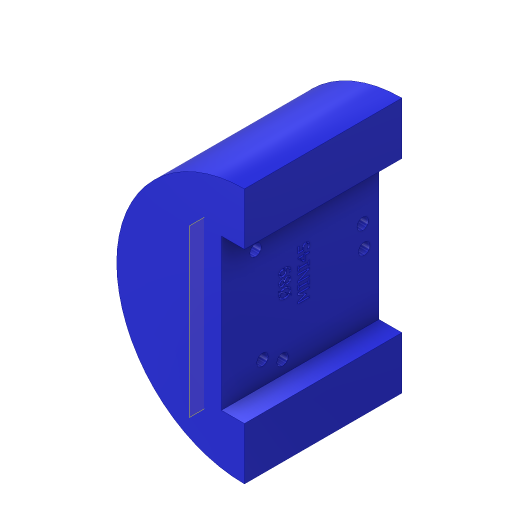
# Autodesk Inventor part: MINI45NewShell89_B
Saved by Autodesk Inventor 2023 (Build 270158000, 158)
## iProperties
Created: 2016-07-01
Part Number: MINI45NewShell89_B
Material: ABS Plastic
Document SubType Name: Modeling
Designer: Administrateur
Density: 1.06 g/cm^3
Appearance: Blue - Wall Paint - Glossy
Author: Administrateur
Autodesk Inventor part; units mm, degrees
ref_plane "XZ Plane" through (0, 0, 0) normal (0, 1, 0) x (-1, 0, 0)
sketch "Sketch1" plane through (0, 0, 0) normal (0, 0, 1) x (1, 0, 0)
  arc A0 (0, 38.9636) -> (0, -38.9636) centre (0, 0) ccw
  line L0 (0, 38.9636) -> (0, 23)
  line L1 (0, 23) -> (-7, 23)
  line L2 (-7, 23) -> (-7, 0)
  line L3 (-46.5484, 0) -> (26.4312, 0) construction
  line L4 (0, -38.9636) -> (0, -23)
  line L5 (0, -23) -> (-7, -23)
  line L6 (-7, -23) -> (-7, 0)
  dimension "d2" = 38.9636
  dimension "d3" = 46
  dimension "d4" = 7
  dimension "d27" = 23
  dimension "d28" = 15.9636
  constraints: 14 end point, 2 horizontal, 2 point on circle, 2 symmetric about line, 1 centre point, 1 coincident, 1 perpendicular, 1 vertical
  measures "d2" radius of A0
  measures "d3" distance between parallel lines of L5 L1
  measures "d4" distance of L0.end L1.end
  measures "d27" distance of L1.end L2.end
  measures "d28" distance of L0.start L0.end
extrude "Extrusion1" add sketch "Sketch1" along normal blind 48
sketch "Sketch2" plane through (-7, -23, 0) normal (1, 0, 0) x (0, 0, -1)
  line L0 (-24, 23) -> (-48, 23) construction
  line L1 (-48, 61.9636) -> (-48, -15.9636) construction
  line L2 (0, 61.9636) -> (-48, 61.9636) construction
  line L3 (-24, 61.9636) -> (-24, -15.9636) construction
  line L4 (0, -15.9636) -> (-48, -15.9636) construction
  line L5 (-24, 23) -> (-37.6292, 37.1134) construction
  circle A0 centre (-24, 23) radius 19.62 construction
  line L6 (-24, 23) -> (-31.9802, 40.9238) construction
  line L7 (-24, 23) -> (-29.408, 4.14) construction
  line L8 (-24, 23) -> (-35.5323, 7.1271) construction
  line L9 (-24, 23) -> (-4.9628, 27.7465) construction
  line L10 (-24, 23) -> (-4.4875, 20.9492) construction
  point P0 (0, 23)
  dimension "d32" = 39.24
  dimension "d34" = 20
  dimension "d37" = 360
  dimension "d39" = 66
  constraints: 16 end point, 11 coincident, 4 midpoint, 2 point on circle, 1 centre point, 17 other
  measures "d32" diameter of A0
  measures "d34" angle of L5 L6
  measures "d39" angle of L0 L6
hole "Hole1" at (-7, 17.9238, 31.9802) at (-7, 14.1134, 37.6292) at (-7, -15.8729, 35.5323) at (-7, -18.86, 29.408) at (-7, -2.0508, 4.4875) at (-7, 4.7465, 4.9628) direction (-1, 0, 0) diameter 3.5 end through all
ref_plane "Work Plane1" through (-38.9636, 0, 0) normal (1, 0, 0) x (0, 1, 0)
ref_plane "Work Plane2" through (-10, 0, 0) normal (1, 0, 0) x (0, 1, 0)
ref_plane "Work Plane3" through (-12.3, -23, 0) normal (1, 0, 0) x (0, 0, -1)
sketch "Sketch4" plane through (-12.3, -23, 0) normal (1, 0, 0) x (0, 0, -1)
  line L0 (0, 61.9636) -> (0, -15.9636) projected
  line L1 (0, -15.9636) -> (-48, -15.9636) projected
  line L2 (-48, 61.9636) -> (-48, -15.9636) projected
  line L3 (0, 61.9636) -> (-48, 61.9636) projected
  circle A0 centre (-31.9802, 40.9238) radius 1.75 projected
  circle A1 centre (-37.6292, 37.1134) radius 1.75 projected
  circle A2 centre (-35.5323, 7.1271) radius 1.75 projected
  circle A3 centre (-29.408, 4.14) radius 1.75 projected
  circle A4 centre (-4.4875, 20.9492) radius 1.75 projected
  circle A5 centre (-4.9628, 27.7465) radius 1.75 projected
  point P0 (0, 23)
  point P1 (-4.4875, 22.6992)
  point P2 (-35.5323, 8.8771)
  point P3 (-31.9802, 42.6738)
  point P4 (-37.6292, 38.8634)
  point P5 (-29.408, 5.89)
  point P6 (-4.9628, 29.4965)
  constraints: 6 coincident, 6 vertical alignment, 6 other
hole "Hole3" at (-12.3, 17.9238, 31.9802) at (-12.3, 14.1134, 37.6292) at (-12.3, -15.8729, 35.5323) at (-12.3, -18.86, 29.408) at (-12.3, -2.0508, 4.4875) at (-12.3, 4.7465, 4.9628) direction (-1, 0, 0) diameter 6.5 end through all
sketch "Sketch6" plane through (-7, -23, 0) normal (1, 0, 0) x (0, 0, -1)
  line L0 (-30.6568, 16.0385) -> (-30.6568, 31.8055) construction
  line L1 (-30.6568, 31.8055) -> (-15.416, 31.8055) construction
  line L2 (-15.416, 31.8055) -> (-15.416, 16.0385) construction
  line L3 (-15.416, 16.0385) -> (-30.6568, 16.0385) construction
  spline S0 degree 2 poles (-28.6913, 22.8428) (-27.8234, 22.8428) (-26.8675, 21.9976) (-26.8675, 21.2942) knots 0 0 0 1 2 2 2
  spline S1 degree 2 poles (-26.8675, 21.2942) (-26.8675, 21.0361) (-27.0037, 20.5908) (-27.1285, 20.4121) knots 0 0 0 1 2 2 2
  line L4 (-27.1285, 20.4121) -> (-26.669, 20.1001)
  line L5 (-26.669, 20.1001) -> (-26.669, 19.7541)
  line L6 (-26.669, 19.7541) -> (-27.3213, 20.1965)
  spline S2 degree 2 poles (-27.3213, 20.1965) (-27.5539, 19.9866) (-28.2403, 19.7484) (-28.6913, 19.7484) knots 0 0 0 1 2 2 2
  spline S3 degree 2 poles (-28.6913, 19.7484) (-29.5563, 19.7484) (-30.515, 20.5964) (-30.515, 21.2942) knots 0 0 0 1 2 2 2
  spline S4 degree 2 poles (-30.515, 21.2942) (-30.515, 21.5636) (-30.3846, 21.9834) (-30.2569, 22.1706) knots 0 0 0 1 2 2 2
  line L7 (-30.2569, 22.1706) -> (-30.6568, 22.44)
  line L8 (-30.6568, 22.44) -> (-30.6568, 22.7889)
  line L9 (-30.6568, 22.7889) -> (-30.0669, 22.3862)
  spline S5 degree 2 poles (-30.0669, 22.3862) (-29.8343, 22.6017) (-29.1593, 22.8428) (-28.6913, 22.8428) knots 0 0 0 1 2 2 2
  spline S6 degree 2 poles (-28.6913, 22.3635) (-29.0146, 22.3635) (-29.5223, 22.233) (-29.6897, 22.1252) knots 0 0 0 1 2 2 2
  line L10 (-29.6897, 22.1252) -> (-27.4858, 20.6503)
  spline S7 degree 2 poles (-27.4858, 20.6503) (-27.3781, 20.7836) (-27.2703, 21.0843) (-27.2703, 21.297) knots 0 0 0 1 2 2 2
  spline S8 degree 2 poles (-27.2703, 21.297) (-27.2703, 21.782) (-28.0021, 22.3635) (-28.6913, 22.3635) knots 0 0 0 1 2 2 2
  spline S9 degree 2 poles (-29.9024, 21.9323) (-30.0073, 21.8104) (-30.1123, 21.4899) (-30.1123, 21.297) knots 0 0 0 1 2 2 2
  spline S10 degree 2 poles (-30.1123, 21.297) (-30.1123, 20.8092) (-29.389, 20.2277) (-28.6913, 20.2277) knots 0 0 0 1 2 2 2
  spline S11 degree 2 poles (-28.6913, 20.2277) (-28.3736, 20.2277) (-27.8801, 20.3497) (-27.7042, 20.4603) knots 0 0 0 1 2 2 2
  line L11 (-27.7042, 20.4603) -> (-29.9024, 21.9323)
  spline S12 degree 2 poles (-26.8619, 24.312) (-26.8619, 24.0511) (-27.0179, 23.6228) (-27.1625, 23.4725) knots 0 0 0 1 2 2 2
  spline S13 degree 2 poles (-27.1625, 23.4725) (-27.3043, 23.325) (-27.6901, 23.1718) (-27.9085, 23.1718) knots 0 0 0 1 2 2 2
  spline S14 degree 2 poles (-27.9085, 23.1718) (-28.1921, 23.1718) (-28.6686, 23.4753) (-28.8104, 23.7646) knots 0 0 0 1 2 2 2
  line L12 (-28.8104, 23.7646) -> (-28.8246, 23.7646)
  spline S15 degree 2 poles (-28.8246, 23.7646) (-28.9749, 23.5065) (-29.3323, 23.2569) (-29.5989, 23.2569) knots 0 0 0 1 2 2 2
  spline S16 degree 2 poles (-29.5989, 23.2569) (-29.9931, 23.2569) (-30.5207, 23.8525) (-30.5207, 24.312) knots 0 0 0 1 2 2 2
  spline S17 degree 2 poles (-30.5207, 24.312) (-30.5207, 24.7885) (-30.0215, 25.3643) (-29.6301, 25.3643) knots 0 0 0 1 2 2 2
  spline S18 degree 2 poles (-29.6301, 25.3643) (-29.3947, 25.3643) (-28.9352, 25.0891) (-28.8047, 24.831) knots 0 0 0 1 2 2 2
  line L13 (-28.8047, 24.831) -> (-28.7905, 24.831)
  spline S19 degree 2 poles (-28.7905, 24.831) (-28.6487, 25.1374) (-28.2403, 25.4522) (-27.917, 25.4522) knots 0 0 0 1 2 2 2
  spline S20 degree 2 poles (-27.917, 25.4522) (-27.4688, 25.4522) (-26.8619, 24.7998) (-26.8619, 24.312) knots 0 0 0 1 2 2 2
  spline S21 degree 2 poles (-27.8716, 24.97) (-28.0871, 24.97) (-28.3424, 24.7998) (-28.4729, 24.5588) knots 0 0 0 1 2 2 2
  spline S22 degree 2 poles (-28.4729, 24.5588) (-28.5183, 24.4793) (-28.6232, 24.2127) (-28.6913, 24.0454) knots 0 0 0 1 2 2 2
  spline S23 degree 2 poles (-28.6913, 24.0454) (-28.5636, 23.8525) (-28.1836, 23.6455) (-27.9425, 23.6455) knots 0 0 0 1 2 2 2
  spline S24 degree 2 poles (-27.9425, 23.6455) (-27.6248, 23.6455) (-27.2107, 24.0284) (-27.2107, 24.3177) knots 0 0 0 1 2 2 2
  spline S25 degree 2 poles (-27.2107, 24.3177) (-27.2107, 24.6126) (-27.5653, 24.97) (-27.8716, 24.97) knots 0 0 0 1 2 2 2
  spline S26 degree 2 poles (-29.6244, 24.9048) (-29.8598, 24.9048) (-30.1747, 24.59) (-30.1747, 24.3092) knots 0 0 0 1 2 2 2
  spline S27 degree 2 poles (-30.1747, 24.3092) (-30.1747, 24.0539) (-29.8939, 23.7277) (-29.6528, 23.7277) knots 0 0 0 1 2 2 2
  spline S28 degree 2 poles (-29.6528, 23.7277) (-29.4798, 23.7277) (-29.2387, 23.8951) (-29.1422, 24.0624) knots 0 0 0 1 2 2 2
  spline S29 degree 2 poles (-29.1422, 24.0624) (-29.1025, 24.1333) (-28.9636, 24.434) (-28.9239, 24.5559) knots 0 0 0 1 2 2 2
  spline S30 degree 2 poles (-28.9239, 24.5559) (-29.0798, 24.7601) (-29.4117, 24.9048) (-29.6244, 24.9048) knots 0 0 0 1 2 2 2
  spline S31 degree 2 poles (-29.3039, 25.784) (-29.5734, 25.784) (-30.0215, 25.9599) (-30.1832, 26.1131) knots 0 0 0 1 2 2 2
  spline S32 degree 2 poles (-30.1832, 26.1131) (-30.3392, 26.2577) (-30.5122, 26.6803) (-30.5122, 26.8959) knots 0 0 0 1 2 2 2
  spline S33 degree 2 poles (-30.5122, 26.8959) (-30.5122, 27.137) (-30.3505, 27.5284) (-30.1974, 27.673) knots 0 0 0 1 2 2 2
  spline S34 degree 2 poles (-30.1974, 27.673) (-30.0045, 27.8545) (-29.3805, 28.0531) (-28.9012, 28.0531) knots 0 0 0 1 2 2 2
  spline S35 degree 2 poles (-28.9012, 28.0531) (-28.4672, 28.0531) (-27.6901, 27.8574) (-27.432, 27.6673) knots 0 0 0 1 2 2 2
  spline S36 degree 2 poles (-27.432, 27.6673) (-27.1597, 27.466) (-26.8732, 26.8987) (-26.8732, 26.4846) knots 0 0 0 1 2 2 2
  spline S37 degree 2 poles (-26.8732, 26.4846) (-26.8732, 26.391) (-26.8931, 26.1783) (-26.9214, 26.0875) knots 0 0 0 1 2 2 2
  line L14 (-26.9214, 26.0875) -> (-27.3724, 26.0875)
  line L15 (-27.3724, 26.0875) -> (-27.3724, 26.1102)
  spline S38 degree 2 poles (-27.3724, 26.1102) (-27.3384, 26.1698) (-27.2788, 26.4194) (-27.2788, 26.547) knots 0 0 0 1 2 2 2
  spline S39 degree 2 poles (-27.2788, 26.547) (-27.2788, 27.0065) (-27.8858, 27.5312) (-28.4474, 27.5681) knots 0 0 0 1 2 2 2
  spline S40 degree 2 poles (-28.4474, 27.5681) (-28.3197, 27.3809) (-28.2034, 27.0405) (-28.2034, 26.8391) knots 0 0 0 1 2 2 2
  spline S41 degree 2 poles (-28.2034, 26.8391) (-28.2034, 26.6463) (-28.2885, 26.3258) (-28.4105, 26.1641) knots 0 0 0 1 2 2 2
  spline S42 degree 2 poles (-28.4105, 26.1641) (-28.5551, 25.9769) (-28.9948, 25.784) (-29.3039, 25.784) knots 0 0 0 1 2 2 2
  spline S43 degree 2 poles (-29.0061, 27.5794) (-29.3606, 27.5794) (-29.8088, 27.449) (-29.9307, 27.3327) knots 0 0 0 1 2 2 2
  spline S44 degree 2 poles (-29.9307, 27.3327) (-30.0442, 27.2306) (-30.1293, 27.0178) (-30.1293, 26.893) knots 0 0 0 1 2 2 2
  spline S45 degree 2 poles (-30.1293, 26.893) (-30.1293, 26.6037) (-29.7152, 26.2605) (-29.3238, 26.2605) knots 0 0 0 1 2 2 2
  spline S46 degree 2 poles (-29.3238, 26.2605) (-29.1025, 26.2605) (-28.8161, 26.374) (-28.714, 26.4988) knots 0 0 0 1 2 2 2
  spline S47 degree 2 poles (-28.714, 26.4988) (-28.6402, 26.5896) (-28.592, 26.8136) (-28.592, 26.9441) knots 0 0 0 1 2 2 2
  spline S48 degree 2 poles (-28.592, 26.9441) (-28.592, 27.0944) (-28.6969, 27.4404) (-28.7849, 27.5709) knots 0 0 0 1 2 2 2
  spline S49 degree 2 poles (-28.7849, 27.5709) (-28.8189, 27.5738) (-28.9352, 27.5794) (-29.0061, 27.5794) knots 0 0 0 1 2 2 2
  line L16 (-21.1786, 19.3938) -> (-21.1786, 18.9287)
  line L17 (-21.1786, 18.9287) -> (-24.1936, 18.9287)
  line L18 (-24.1936, 18.9287) -> (-22.143, 18.0154)
  line L19 (-22.143, 18.0154) -> (-22.143, 17.7318)
  line L20 (-22.143, 17.7318) -> (-24.1936, 16.827)
  line L21 (-24.1936, 16.827) -> (-21.1786, 16.827)
  line L22 (-21.1786, 16.827) -> (-21.1786, 16.393)
  line L23 (-21.1786, 16.393) -> (-24.6786, 16.393)
  line L24 (-24.6786, 16.393) -> (-24.6786, 17.0284)
  line L25 (-24.6786, 17.0284) -> (-22.7301, 17.902)
  line L26 (-22.7301, 17.902) -> (-24.6786, 18.7472)
  line L27 (-24.6786, 18.7472) -> (-24.6786, 19.3938)
  line L28 (-24.6786, 19.3938) -> (-21.1786, 19.3938)
  line L29 (-21.1786, 21.3225) -> (-21.1786, 19.9668)
  line L30 (-21.1786, 19.9668) -> (-21.536, 19.9668)
  line L31 (-21.536, 19.9668) -> (-21.536, 20.4121)
  line L32 (-21.536, 20.4121) -> (-24.3212, 20.4121)
  line L33 (-24.3212, 20.4121) -> (-24.3212, 19.9668)
  line L34 (-24.3212, 19.9668) -> (-24.6786, 19.9668)
  line L35 (-24.6786, 19.9668) -> (-24.6786, 21.3225)
  line L36 (-24.6786, 21.3225) -> (-24.3212, 21.3225)
  line L37 (-24.3212, 21.3225) -> (-24.3212, 20.8772)
  line L38 (-24.3212, 20.8772) -> (-21.536, 20.8772)
  line L39 (-21.536, 20.8772) -> (-21.536, 21.3225)
  line L40 (-21.536, 21.3225) -> (-21.1786, 21.3225)
  line L41 (-21.1786, 24.4028) -> (-21.1786, 23.8809)
  line L42 (-21.1786, 23.8809) -> (-24.1964, 22.3323)
  line L43 (-24.1964, 22.3323) -> (-21.1786, 22.3323)
  line L44 (-21.1786, 22.3323) -> (-21.1786, 21.8983)
  line L45 (-21.1786, 21.8983) -> (-24.6786, 21.8983)
  line L46 (-24.6786, 21.8983) -> (-24.6786, 22.5592)
  line L47 (-24.6786, 22.5592) -> (-21.9075, 23.9688)
  line L48 (-21.9075, 23.9688) -> (-24.6786, 23.9688)
  line L49 (-24.6786, 23.9688) -> (-24.6786, 24.4028)
  line L50 (-24.6786, 24.4028) -> (-21.1786, 24.4028)
  line L51 (-21.1786, 26.3314) -> (-21.1786, 24.9757)
  line L52 (-21.1786, 24.9757) -> (-21.536, 24.9757)
  line L53 (-21.536, 24.9757) -> (-21.536, 25.421)
  line L54 (-21.536, 25.421) -> (-24.3212, 25.421)
  line L55 (-24.3212, 25.421) -> (-24.3212, 24.9757)
  line L56 (-24.3212, 24.9757) -> (-24.6786, 24.9757)
  line L57 (-24.6786, 24.9757) -> (-24.6786, 26.3314)
  line L58 (-24.6786, 26.3314) -> (-24.3212, 26.3314)
  line L59 (-24.3212, 26.3314) -> (-24.3212, 25.8861)
  line L60 (-24.3212, 25.8861) -> (-21.536, 25.8861)
  line L61 (-21.536, 25.8861) -> (-21.536, 26.3314)
  line L62 (-21.536, 26.3314) -> (-21.1786, 26.3314)
  line L63 (-22.3812, 29.06) -> (-22.3812, 28.643)
  line L64 (-22.3812, 28.643) -> (-21.1786, 28.643)
  line L65 (-21.1786, 28.643) -> (-21.1786, 28.1921)
  line L66 (-21.1786, 28.1921) -> (-22.3812, 28.1921)
  line L67 (-22.3812, 28.1921) -> (-22.3812, 26.6463)
  line L68 (-22.3812, 26.6463) -> (-22.8747, 26.6463)
  line L69 (-22.8747, 26.6463) -> (-24.6786, 28.2119)
  line L70 (-24.6786, 28.2119) -> (-24.6786, 28.643)
  line L71 (-24.6786, 28.643) -> (-22.7584, 28.643)
  line L72 (-22.7584, 28.643) -> (-22.7584, 29.06)
  line L73 (-22.7584, 29.06) -> (-22.3812, 29.06)
  line L74 (-22.7584, 28.1921) -> (-24.1255, 28.1921)
  line L75 (-24.1255, 28.1921) -> (-22.7584, 27.015)
  line L76 (-22.7584, 27.015) -> (-22.7584, 28.1921)
  spline S50 degree 2 poles (-22.2905, 31.5559) (-22.038, 31.5559) (-21.6069, 31.3943) (-21.4481, 31.2468) knots 0 0 0 1 2 2 2
  spline S51 degree 2 poles (-21.4481, 31.2468) (-21.2892, 31.0993) (-21.1049, 30.6597) (-21.1049, 30.3874) knots 0 0 0 1 2 2 2
  spline S52 degree 2 poles (-21.1049, 30.3874) (-21.1049, 30.1378) (-21.2155, 29.6499) (-21.3034, 29.4712) knots 0 0 0 1 2 2 2
  line L77 (-21.3034, 29.4712) -> (-21.7998, 29.4712)
  line L78 (-21.7998, 29.4712) -> (-21.7998, 29.5053)
  spline S53 degree 2 poles (-21.7998, 29.5053) (-21.7601, 29.5592) (-21.658, 29.7605) (-21.6126, 29.8825) knots 0 0 0 1 2 2 2
  spline S54 degree 2 poles (-21.6126, 29.8825) (-21.5644, 30.0215) (-21.5105, 30.2512) (-21.5105, 30.3959) knots 0 0 0 1 2 2 2
  spline S55 degree 2 poles (-21.5105, 30.3959) (-21.5105, 30.5377) (-21.6126, 30.8043) (-21.7232, 30.9007) knots 0 0 0 1 2 2 2
  spline S56 degree 2 poles (-21.7232, 30.9007) (-21.8281, 30.9887) (-22.1061, 31.0794) (-22.2933, 31.0794) knots 0 0 0 1 2 2 2
  spline S57 degree 2 poles (-22.2933, 31.0794) (-22.4805, 31.0794) (-22.7187, 30.9773) (-22.7981, 30.8809) knots 0 0 0 1 2 2 2
  spline S58 degree 2 poles (-22.7981, 30.8809) (-22.8861, 30.7816) (-22.9598, 30.4866) (-22.9598, 30.3079) knots 0 0 0 1 2 2 2
  spline S59 degree 2 poles (-22.9598, 30.3079) (-22.9598, 30.1151) (-22.9003, 29.7322) (-22.8747, 29.6159) knots 0 0 0 1 2 2 2
  line L79 (-22.8747, 29.6159) -> (-24.6786, 29.6159)
  line L80 (-24.6786, 29.6159) -> (-24.6786, 31.5361)
  line L81 (-24.6786, 31.5361) -> (-24.2674, 31.5361)
  line L82 (-24.2674, 31.5361) -> (-24.2674, 30.0669)
  line L83 (-24.2674, 30.0669) -> (-23.3342, 30.0669)
  spline S60 degree 2 poles (-23.3342, 30.0669) (-23.3456, 30.152) (-23.3541, 30.3165) (-23.3541, 30.3845) knots 0 0 0 1 2 2 2
  spline S61 degree 2 poles (-23.3541, 30.3845) (-23.3541, 30.654) (-23.2661, 31.0255) (-23.1357, 31.1957) knots 0 0 0 1 2 2 2
  spline S62 degree 2 poles (-23.1357, 31.1957) (-23.0052, 31.3687) (-22.6081, 31.5559) (-22.2905, 31.5559) knots 0 0 0 1 2 2 2
  point P0 (0, 23)
  constraints: 2 other
extrude "Extrusion3" cut sketch "Sketch6" against normal blind 1
equation "\"d27\" = 0.5 * d3"
equation "\"d28\" = -0.5 * d3 + d2"
body "Solid1"
